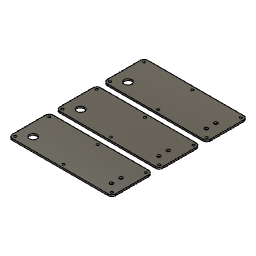
Back Panel 3x (Autodesk Fusion 360 design; units mm, degrees)
Autodesk Fusion 360 part; units mm, degrees
sketch "Main Body" plane through (0, 0, 0) normal (0, 0, 1) x (1, 0, 0)
  line L0 (50.5, 21.5) -> (-50.5, 21.5)
  line L1 (-54.5, 17.5) -> (-54.5, -17.5)
  line L2 (-50.5, -21.5) -> (50.5, -21.5)
  line L3 (54.5, -17.5) -> (54.5, 17.5)
  arc A0 (-50.5, 21.5) -> (-54.5, 17.5) centre (-50.5, 17.5) ccw
  arc A1 (-54.5, -17.5) -> (-50.5, -21.5) centre (-50.5, -17.5) ccw
  arc A2 (50.5, -21.5) -> (54.5, -17.5) centre (50.5, -17.5) ccw
  arc A3 (54.5, 17.5) -> (50.5, 21.5) centre (50.5, 17.5) ccw
  line L4 (-54.5, 0) -> (54.5, 0) construction
  line L5 (0, 21.5) -> (0, -21.5) construction
  dimension "d3" = 4
  dimension "d4" = 4
  dimension "d5" = 4
  dimension "d6" = 4
  dimension "d7" = 109
  dimension "d8" = 43
  constraint horizontal L0
  constraint perpendicular L0 L1
  constraint parallel L0 L2
  constraint parallel L1 L3
  constraint tangent L0 A0
  constraint tangent L1 A0
  constraint tangent L1 A1
  constraint tangent L2 A1
  constraint tangent L2 A2
  constraint tangent L3 A2
  constraint tangent L3 A3
  constraint tangent L0 A3
  constraint horizontal L4
  constraint midpoint L3 L4.end
  constraint coincident L1 L4.start
  constraint vertical L5
  constraint midpoint origin L4
  constraint midpoint L0 L5.start
  constraint midpoint origin L5
  measures "d3" radius of A0
  measures "d4" radius of A1
  measures "d5" radius of A2
  measures "d6" radius of A3
  measures "d7" distance of L4.start L4.end
  measures "d8" distance of L5.start L5.end
extrude "Extrude1" add sketch "Main Body" along normal blind 1.6 makes body 1
sketch "Screw Holes" plane through (0, 0, 1.6) normal (0, 0, 1) x (-1, 0, 0)
  arc A0 (-54.5, -17.5) -> (-50.5, -21.5) centre (-50.5, -17.5) ccw
  line L0 (-50.5, -21.5) -> (50.5, -21.5)
  arc A1 (50.5, -21.5) -> (54.5, -17.5) centre (50.5, -17.5) ccw
  line L1 (54.5, -17.5) -> (54.5, 17.5)
  arc A2 (54.5, 17.5) -> (50.5, 21.5) centre (50.5, 17.5) ccw
  line L2 (50.5, 21.5) -> (-50.5, 21.5)
  arc A3 (-50.5, 21.5) -> (-54.5, 17.5) centre (-50.5, 17.5) ccw
  line L3 (-54.5, 17.5) -> (-54.5, -17.5)
  circle A4 centre (-51, 18) radius 1.19
  line L4 (51, 0) -> (-51, 0) construction
  line L5 (0, -18) -> (0, 18) construction
  line L6 (-51, -18) -> (-51, 18) construction
  line L7 (51, -18) -> (51, 18) construction
  circle A5 centre (-51, -18) radius 1.19
  circle A6 centre (0, 18) radius 1.19
  circle A7 centre (0, -18) radius 1.19
  circle A8 centre (51, -18) radius 1.19
  circle A9 centre (51, 18) radius 1.19
  dimension "d11" = 2.38
  dimension "d12" = 102
  dimension "d13" = 36
  dimension "d14" = 36
  dimension "d15" = 36
  dimension "d16" = 2.38
  dimension "d17" = 2.38
  dimension "d18" = 2.38
  dimension "d19" = 2.38
  dimension "d20" = 2.38
  constraint horizontal L4
  constraint midpoint origin L4
  constraint vertical L5
  constraint vertical L6
  constraint vertical L7
  constraint midpoint L4.start L7
  constraint midpoint origin L5
  constraint midpoint L4.end L6
  constraint coincident L7.end A9.centre
  constraint coincident L7.start A8.centre
  constraint coincident L5.start A7.centre
  constraint coincident L5.end A6.centre
  constraint coincident A4.centre L6.end
  constraint coincident L6.start A5.centre
  measures "d11" diameter of A4
  measures "d12" distance of L4.start L4.end
  measures "d13" distance of L5.start L5.end
  measures "d14" distance of L6.start A4.centre
  measures "d15" distance of L7.start L7.end
  measures "d16" diameter of A5
  measures "d17" diameter of A6
  measures "d18" diameter of A7
  measures "d19" diameter of A8
  measures "d20" diameter of A9
extrude "Extrude2" cut sketch "Screw Holes" against normal blind 1.6 contours A4 | A5 | A6 | A7 | A8 | A9 bodies 1
sketch "Button Holes" plane through (0, 0, 1.6) normal (0, 0, 1) x (-1, 0, 0)
  circle A0 centre (0, 18) radius 1.19
  circle A1 centre (0, -18) radius 1.19
  circle A2 centre (51, -18) radius 1.19
  circle A3 centre (-51, 18) radius 1.19
  circle A4 centre (-51, -18) radius 1.19
  circle A5 centre (51, 18) radius 1.19
  arc A6 (-54.5, -17.5) -> (-50.5, -21.5) centre (-50.5, -17.5) ccw
  line L0 (-50.5, -21.5) -> (50.5, -21.5)
  arc A7 (50.5, -21.5) -> (54.5, -17.5) centre (50.5, -17.5) ccw
  line L1 (54.5, -17.5) -> (54.5, 17.5)
  arc A8 (54.5, 17.5) -> (50.5, 21.5) centre (50.5, 17.5) ccw
  line L2 (50.5, 21.5) -> (-50.5, 21.5)
  arc A9 (-50.5, 21.5) -> (-54.5, 17.5) centre (-50.5, 17.5) ccw
  line L3 (-54.5, 17.5) -> (-54.5, -17.5)
  line L4 (-42.65, 0.05) -> (-42.65, 10.05) construction
  circle A10 centre (-42.65, 0.05) radius 1.75
  circle A11 centre (-42.65, 10.05) radius 1.75
  line L5 (0, 0) -> (-42.65, 0) construction
  line L6 (-42.65, 0) -> (-42.65, 0.05)
  dimension "d23" = 10
  dimension "d24" = 3.5
  dimension "d25" = 3.5
  dimension "d26" = 42.65
  dimension "d27" = 0.05
  constraint vertical L4
  constraint coincident L4.start A10.centre
  constraint coincident L4.end A11.centre
  constraint coincident L5.start origin
  constraint horizontal L5
  constraint vertical L6
  measures "d23" distance of L4.start L4.end
  measures "d24" diameter of A10
  measures "d25" diameter of A11
  measures "d26" distance of L5.start L5.end
  measures "d27" distance of L5.end L4.start
extrude "Extrude3" cut sketch "Button Holes" against normal blind 1.6 contours A10 | A11 bodies 1
sketch "Power Jack Hole" plane through (0, 0, 1.6) normal (0, 0, 1) x (-1, 0, 0)
  circle A0 centre (-42.65, 0.05) radius 1.75
  circle A1 centre (-42.65, 10.05) radius 1.75
  circle A2 centre (0, 18) radius 1.19
  circle A3 centre (0, -18) radius 1.19
  circle A4 centre (51, -18) radius 1.19
  circle A5 centre (-51, 18) radius 1.19
  circle A6 centre (-51, -18) radius 1.19
  circle A7 centre (51, 18) radius 1.19
  arc A8 (-54.5, -17.5) -> (-50.5, -21.5) centre (-50.5, -17.5) ccw
  line L0 (-50.5, -21.5) -> (50.5, -21.5)
  arc A9 (50.5, -21.5) -> (54.5, -17.5) centre (50.5, -17.5) ccw
  line L1 (54.5, -17.5) -> (54.5, 17.5)
  arc A10 (54.5, 17.5) -> (50.5, 21.5) centre (50.5, 17.5) ccw
  line L2 (50.5, 21.5) -> (-50.5, 21.5)
  arc A11 (-50.5, 21.5) -> (-54.5, 17.5) centre (-50.5, 17.5) ccw
  line L3 (-54.5, 17.5) -> (-54.5, -17.5)
  line L4 (0, 0) -> (41.3, 0) construction
  line L5 (41.3, 0) -> (41.3, 8.7) construction
  circle A12 centre (41.3, 8.7) radius 4.05
  dimension "d30" = 41.3
  dimension "d31" = 8.7
  dimension "d32" = 8.1
  constraint horizontal L4
  constraint coincident L4.start origin
  constraint vertical L5
  constraint coincident L4.end L5.start
  constraint coincident L5.end A12.centre
  measures "d30" distance of L4.start L4.end
  measures "d31" distance of L4.end L5.end
  measures "d32" diameter of A12
extrude "Extrude4" cut sketch "Power Jack Hole" against normal blind 1.6 contours A12 bodies 1
copy_body "CopyPasteBodies1" bodies 1 makes body 2
move_body "Move1" bodies 2 to x (1, 0, 0) y (0, 1, 0) z (0, 0, 1) at (0, -50, 0)
copy_body "CopyPasteBodies2" bodies 2 makes body 3
move_body "Move2" bodies 3 to x (1, 0, 0) y (0, 1, 0) z (0, 0, 1) at (0, -50, 0)
